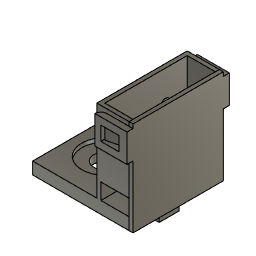
bumper_end (Autodesk Fusion 360 design; units mm, degrees)
Autodesk Fusion 360 part; units mm, degrees
sketch "Sketch1" plane through (0, 0, 0) normal (0, 0, 1) x (1, 0, 0) in component "Halterung"
  line L0 (0, 0) -> (24, 0)
  line L1 (24, 0) -> (24, 20)
  line L2 (24, 20) -> (0, 20)
  line L3 (0, 20) -> (0, 0)
  dimension "d1" = 20
  dimension "d2" = 24
  constraint horizontal L0
  constraint vertical L1
  constraint horizontal L2
  constraint vertical L3
  constraint coincident L0.start L3.end
  measures "d1" distance of L0.start L2.end
  measures "d2" distance of L0.start L0.end
extrude "Extrude1" add sketch "Sketch1" along normal blind 3 makes body 1 in component "Halterung"
sketch "Anbohrung" plane through (0, 0, 3) normal (0, 0, 1) x (-1, 0, 0) in component "Halterung"
  line L0 (0, -20) -> (0, 0)
  line L1 (0, 0) -> (-24, 0)
  line L2 (-24, 0) -> (-24, -20)
  line L3 (-24, -20) -> (0, -20)
  circle A0 centre (-8, -10) radius 5.75
  dimension "d5" = 11.5
  dimension "d6" = 10
  dimension "d21" = 8
  dimension "d22" = 2.25
  measures "d5" diameter of A0
  measures "d6" distance of L3 A0.centre
  measures "d21" distance of L0 A0.centre
  measures "d22" distance of L0 A0
extrude "Extrude2" cut sketch "Anbohrung" against normal blind 1 contours A0 bodies 1 in component "Halterung"
sketch "Bohrloch" plane through (0, 0, 2) normal (0, 0, 1) x (-1, 0, 0) in component "Halterung"
  circle A0 centre (-8, -10) radius 2.75
  circle A1 centre (-8, -10) radius 5.75
  dimension "d10" = 5.5
  constraint concentric A0 A1
  measures "d10" diameter of A0
extrude "Extrude3" cut sketch "Bohrloch" against normal up to surface (2 mm away) contours A0 bodies 1 in component "Halterung"
sketch "Horizontale Halterung" plane through (0, 0, 0) normal (0, 0, -1) x (1, 0, 0) in component "Halterung"
  circle A0 centre (8, -10) radius 2.75
  line L0 (0, 0) -> (0, -20)
  line L1 (0, -20) -> (24, -20)
  line L2 (24, -20) -> (24, 0)
  line L3 (24, 0) -> (0, 0)
  line L4 (24, -7.5) -> (21, -7.5)
  line L5 (24, -12.5) -> (24, -7.5)
  line L6 (21, -12.5) -> (24, -12.5)
  line L7 (21, -7.5) -> (21, -12.5)
  dimension "d44" = 3
  dimension "d45" = 5
  dimension "d46" = 7.5
  constraint collinear L2 L5
  constraint equal L5 L7
  constraint equal L4 L6
  measures "d44" distance of L4.start L4.end
  measures "d45" distance of L4.end L6.start
  measures "d46" distance of L3 L4
extrude "Extrude4" add sketch "Horizontale Halterung" along normal blind 2 contours L2 L4 L5 L6 L7 bodies 1 in component "Halterung"
sketch "Haltearm" plane through (0, 0, 3) normal (0, 0, 1) x (-1, 0, 0) in component "Halterung"
  line L0 (0, -20) -> (0, 0)
  line L1 (0, 0) -> (-24, 0)
  line L2 (-24, 0) -> (-24, -20)
  line L3 (-24, -20) -> (0, -20)
  line L4 (-24, -20) -> (-16, -20)
  line L5 (-16, -20) -> (-16, 0)
  line L6 (-16, 0) -> (-24, 0)
  line L7 (-24, 0) -> (-24, -20)
  circle A0 centre (-8, -10) radius 5.75
  dimension "d18" = 8
  constraint horizontal L4
  constraint vertical L5
  constraint horizontal L6
  constraint vertical L7
  constraint coincident L2.end L3.start
  measures "d18" distance of L2.end L4.end
extrude "Extrude6" add sketch "Haltearm" along normal blind 20.5 contours L1 L2 L3 L4 L5 L6 L7 bodies 1 in component "Halterung"
sketch "Hoehenerweiterung" plane through (0, 20, 0) normal (0, 1, 0) x (-1, 0, 0) in component "Halterung"
  line L0 (-24, 0) -> (0, 0)
  line L1 (0, 0) -> (0, 3)
  line L2 (0, 3) -> (-16, 3)
  line L3 (-16, 3) -> (-16, 23.5)
  line L4 (-16, 23.5) -> (-24, 23.5)
  line L5 (-24, 23.5) -> (-24, 0)
  line L6 (-16, 23.5) -> (-24, 23.5)
  line L7 (-24, 23.5) -> (-24, 0)
  line L8 (-24, 0) -> (-16, 0)
  line L9 (-16, 0) -> (-16, 23.5)
  constraint horizontal L6
  constraint vertical L7
  constraint horizontal L8
  constraint vertical L9
  constraint coincident L0.start L5.end
  constraint coincident L3.end L4.start
extrude "Extrude7" add sketch "Hoehenerweiterung" along normal blind 2.5 contours L0 L3 L4 L5 L6 L7 L8 L9 bodies 1 in component "Halterung"
sketch "Aushoelung" plane through (0, 0, 23.5) normal (0, 0, 1) x (-1, 0, 0) in component "Halterung"
  line L0 (-24, 0) -> (-24, -22.5)
  line L1 (-24, -22.5) -> (-16, -22.5)
  line L2 (-16, -22.5) -> (-16, 0)
  line L3 (-16, 0) -> (-24, 0)
  line L4 (-17, -21.5) -> (-24, -21.5)
  line L5 (-24, -21.5) -> (-24, -1)
  line L6 (-24, -1) -> (-17, -1)
  line L7 (-17, -1) -> (-17, -21.5)
  dimension "d27" = 1
  dimension "d28" = 1
  dimension "d29" = 1
  constraint horizontal L4
  constraint vertical L5
  constraint horizontal L6
  constraint vertical L7
  constraint collinear L0 L5
  measures "d27" distance of L1 L4
  measures "d28" distance of L3 L6
  measures "d29" distance of L2 L7
extrude "Extrude8" cut sketch "Aushoelung" against normal up to surface (20.5 mm away) contours L0 L4 L5 L6 L7 bodies 1 in component "Halterung"
sketch "Servoarme" plane through (17, 0, 0) normal (1, 0, 0) x (0, 1, 0) in component "Halterung"
  line L0 (1, 3) -> (21.5, 3)
  line L1 (21.5, 3) -> (21.5, 23.5)
  line L2 (21.5, 23.5) -> (1, 23.5)
  line L3 (1, 23.5) -> (1, 3)
  circle A0 centre (16.1, 15.9) radius 1.1
  circle A1 centre (6.4, 15.9) radius 1.1
  dimension "d32" = 2.2
  dimension "d34" = 4
  dimension "d35" = 4.3
  dimension "d36" = 6.5
  dimension "d37" = 6.5
  dimension "d40" = 7.5
  constraint equal A0 A1
  measures "d32" diameter of A0
  measures "d35" distance of L3 A1
  measures "d36" distance of L2 A1
  measures "d37" distance of L2 A0
  measures "d40" distance of A0 A1
extrude "Extrude9" add sketch "Servoarme" along normal up to surface (7.5 mm away) contours A0 | A1 bodies 1 in component "Halterung"
sketch "Kabeloeffnung" plane through (0, 1, 0) normal (0, 1, 0) x (-1, 0, 0) in component "Halterung"
  line L0 (-24, 3) -> (-17, 3)
  line L1 (-17, 3) -> (-17, 23.5)
  line L2 (-17, 23.5) -> (-24, 23.5)
  line L3 (-24, 23.5) -> (-24, 3)
  line L4 (-24, 3) -> (-17, 3)
  line L5 (-17, 3) -> (-17, 7)
  line L6 (-17, 7) -> (-24, 7)
  line L7 (-24, 7) -> (-24, 3)
  dimension "d41" = 4
  constraint horizontal L4
  constraint vertical L5
  constraint horizontal L6
  constraint vertical L7
  constraint coincident L1 L5.end
  constraint coincident L0.start L3.end
  measures "d41" distance of L0.start L6.end
extrude "Extrude10" cut sketch "Kabeloeffnung" against normal up to surface (1 mm away) contours L0 L1 L3 L4 L5 L6 L7 bodies 1 in component "Halterung"
sketch "Clip" plane through (0, 0, 0) normal (0, -1, 0) x (1, 0, 0) in component "Halterung"
  line L0 (24, 3) -> (17, 3)
  line L1 (17, 3) -> (17, 7)
  line L2 (17, 7) -> (24, 7)
  line L3 (24, 7) -> (24, 23.5)
  line L4 (24, 23.5) -> (16, 23.5)
  line L5 (16, 23.5) -> (16, 3)
  line L6 (16, 3) -> (0, 3)
  line L7 (0, 3) -> (0, 0)
  line L8 (0, 0) -> (24, 0)
  line L9 (24, 0) -> (24, 3)
  line L10 (19, 20.5) -> (23, 20.5)
  line L11 (23, 20.5) -> (23, 17.5)
  line L12 (23, 17.5) -> (19, 17.5)
  line L13 (19, 17.5) -> (19, 20.5)
  dimension "d48" = 3
  dimension "d49" = 3
  dimension "d50" = 1
  dimension "d52" = 4
  constraint horizontal L10
  constraint vertical L11
  constraint horizontal L12
  constraint vertical L13
  measures "d48" distance of L10.end L11.end
  measures "d49" distance of L4 L10
  measures "d50" distance of L3 L11
  measures "d52" distance of L10.start L10.end
extrude "Extrude11" add sketch "Clip" along normal blind 1 contours L10 L11 L12 L13 bodies 1 in component "Halterung"
chamfer "Chamfer1" distance 4 distance2 1 1 edges at (23, -1, 19) measured on face at (21.6667, -1, 18.5) on bodies 1 in component "Halterung"
sketch "Clip (1)" plane through (0, 22.5, 0) normal (0, 1, 0) x (-1, 0, 0) in component "Halterung"
  line L0 (-16, 0) -> (-16, 23.5)
  line L1 (-16, 23.5) -> (-24, 23.5)
  line L2 (-24, 23.5) -> (-24, 0)
  line L3 (-24, 0) -> (-16, 0)
  line L4 (-23, 20.5) -> (-19, 20.5)
  line L5 (-19, 20.5) -> (-19, 17.5)
  line L6 (-19, 17.5) -> (-23, 17.5)
  line L7 (-23, 17.5) -> (-23, 20.5)
  dimension "d59" = 3
  dimension "d60" = 3
  dimension "d71" = 4
  dimension "d72" = 1
  constraint horizontal L4
  constraint vertical L5
  constraint horizontal L6
  constraint vertical L7
  measures "d59" distance of L4.end L5.end
  measures "d60" distance of L1 L4
  measures "d71" distance of L4.start L4.end
  measures "d72" distance of L2 L7
extrude "Extrude12" add sketch "Clip (1)" along normal blind 1 contours L4 L5 L6 L7 bodies 1 in component "Halterung"
chamfer "Chamfer2" distance 4 distance2 1 1 edges at (23, 23.5, 19) measured on face at (21.6667, 23.5, 19.5) on bodies 1 in component "Halterung"
sketch "Klappe" plane through (24, 0, 0) normal (1, 0, 0) x (0, 1, 0) in component "Klappe"
  line L0 (21.5, 3) -> (0, 3)
  line L1 (0, 3) -> (0, 0)
  line L2 (0, 0) -> (7.5, 0)
  line L3 (7.5, 0) -> (7.5, -2)
  line L4 (7.5, -2) -> (12.5, -2)
  line L5 (12.5, -2) -> (12.5, 0)
  line L6 (12.5, 0) -> (22.5, 0)
  line L7 (22.5, 0) -> (22.5, 23.5)
  line L8 (22.5, 23.5) -> (21.5, 23.5)
  line L9 (21.5, 23.5) -> (21.5, 3)
  line L10 (0, 0) -> (22.5, 0)
  line L11 (22.5, 0) -> (22.5, 23.5)
  line L12 (22.5, 23.5) -> (0, 23.5)
  line L13 (0, 23.5) -> (0, 0)
  constraint horizontal L10
  constraint vertical L11
  constraint horizontal L12
  constraint vertical L13
  constraint coincident L7.end L8.start
  constraint coincident L1.end L2.start
extrude "Extrude1'" add sketch "Klappe" along normal blind 1 separate body contours L0 L1 L2 L6 L7 L8 L9 L10 L11 L12 L13 | L0 L9 L12 L13 makes body 2 in component "Klappe"
extrude "Extrude13" [suppressed] in component "Halterung"
extrude "Extrude2'" cut 2 faces at (24.5, 6.534, 16.3506) (24.5, 16.4463, 15.8466) along direction (-1, 0, 0) blind 0.5 on bodies 1 bodies 2 in component "Klappe"
sketch "Sketch2" plane through (0, 0, 0) normal (0, -1, 0) x (1, 0, 0) in component "Klappe"
  line L0 (24, 23.5) -> (24, 0)
  line L1 (24, 0) -> (25, 0)
  line L2 (25, 0) -> (25, 23.5)
  line L3 (25, 23.5) -> (24, 23.5)
  line L4 (24, 22.5) -> (25, 22.5)
  line L5 (25, 22.5) -> (25, 15.5)
  line L6 (25, 15.5) -> (24, 15.5)
  line L7 (24, 15.5) -> (24, 22.5)
  dimension "d73" = 1
  dimension "d74" = 7
  constraint horizontal L4
  constraint vertical L5
  constraint horizontal L6
  constraint vertical L7
  constraint coincident L2 L5.end
  constraint coincident L0 L4.start
  measures "d73" distance of L3 L4
  measures "d74" distance of L4.end L5.end
extrude "Extrude3'" add sketch "Sketch2" along normal blind 1.5 contours L0 L2 L4 L5 L6 L7 bodies 2 in component "Klappe"
sketch "Sketch3" plane through (0, 22.5, 0) normal (0, 1, 0) x (-1, 0, 0) in component "Klappe"
  line L0 (-24, 0) -> (-24, 23.5)
  line L1 (-24, 23.5) -> (-25, 23.5)
  line L2 (-25, 23.5) -> (-25, 0)
  line L3 (-25, 0) -> (-24, 0)
  line L4 (-25, 22.5) -> (-24, 22.5)
  line L5 (-24, 22.5) -> (-24, 15.5)
  line L6 (-24, 15.5) -> (-25, 15.5)
  line L7 (-25, 15.5) -> (-25, 22.5)
  dimension "d77" = 1
  dimension "d78" = 7
  constraint horizontal L4
  constraint vertical L5
  constraint horizontal L6
  constraint vertical L7
  constraint coincident L0 L5.end
  constraint coincident L2 L4.start
  measures "d77" distance of L1 L4
  measures "d78" distance of L4.start L6.end
extrude "Extrude4'" add sketch "Sketch3" along normal blind 1.5 contours L0 L2 L4 L5 L6 L7 bodies 2 in component "Klappe"
sketch "Sketch4" plane through (24, 0, 0) normal (-1, 0, 0) x (0, -1, 0) in component "Klappe"
  circle A0 centre (-6.4, 15.9) radius 1.1
  circle A1 centre (-16.1, 15.9) radius 1.1
  line L0 (0, 22.5) -> (0, 23.5)
  line L1 (0, 23.5) -> (-22.5, 23.5)
  line L2 (-22.5, 23.5) -> (-22.5, 22.5)
  line L3 (-22.5, 22.5) -> (-24, 22.5)
  line L4 (-24, 22.5) -> (-24, 15.5)
  line L5 (-24, 15.5) -> (-22.5, 15.5)
  line L6 (-22.5, 15.5) -> (-22.5, 0)
  line L7 (-22.5, 0) -> (0, 0)
  line L8 (0, 0) -> (0, 15.5)
  line L9 (0, 15.5) -> (1.5, 15.5)
  line L10 (1.5, 15.5) -> (1.5, 22.5)
  line L11 (1.5, 22.5) -> (0, 22.5)
  line L12 (-24, 22.5) -> (-22.5, 22.5)
  line L13 (-22.5, 22.5) -> (-22.5, 15.5)
  line L14 (-22.5, 15.5) -> (-24, 15.5)
  line L15 (-24, 15.5) -> (-24, 22.5)
  line L16 (0, 22.5) -> (1.5, 22.5)
  line L17 (1.5, 22.5) -> (1.5, 15.5)
  line L18 (1.5, 15.5) -> (0, 15.5)
  line L19 (0, 15.5) -> (0, 22.5)
  constraint horizontal L12
  constraint vertical L13
  constraint horizontal L14
  constraint vertical L15
  constraint coincident L5.end L6.start
  constraint coincident L3.end L4.start
  constraint horizontal L16
  constraint vertical L17
  constraint horizontal L18
  constraint vertical L19
  constraint coincident L9.end L10.start
  constraint coincident L0.start L11.end
extrude "Extrude5" add sketch "Sketch4" along normal blind 7 contours L9 L10 L11 L16 L17 L18 L19 | L3 L4 L5 L12 L13 L14 L15 bodies 2 in component "Klappe"
sketch "Sketch5" plane through (0, 24, 0) normal (0, 1, 0) x (-1, 0, 0) in component "Klappe"
  line L0 (-25, 15.5) -> (-17, 15.5)
  line L1 (-17, 15.5) -> (-17, 22.5)
  line L2 (-17, 22.5) -> (-25, 22.5)
  line L3 (-25, 22.5) -> (-25, 15.5)
  line L4 (-18.5, 20.75) -> (-23, 20.75)
  line L5 (-23, 20.75) -> (-23, 17.25)
  line L6 (-23, 17.25) -> (-18.5, 17.25)
  line L7 (-18.5, 17.25) -> (-18.5, 20.75)
  dimension "d83" = 3.5
  dimension "d84" = 4.5
  dimension "d85" = 1.75
  dimension "d97" = 2
  constraint horizontal L4
  constraint vertical L5
  constraint horizontal L6
  constraint vertical L7
  measures "d83" distance of L4.start L6.end
  measures "d84" distance of L4.start L4.end
  measures "d85" distance of L2 L4
  measures "d97" distance of L3 L5
extrude "Extrude6'" cut sketch "Sketch5" against normal up to surface (1.5 mm away) contours L4 L5 L6 L7 bodies 2 in component "Klappe"
sketch "Sketch6" plane through (0, -1.5, 0) normal (0, -1, 0) x (1, 0, 0) in component "Klappe"
  line L0 (17, 15.5) -> (25, 15.5)
  line L1 (25, 15.5) -> (25, 22.5)
  line L2 (25, 22.5) -> (17, 22.5)
  line L3 (17, 22.5) -> (17, 15.5)
  line L4 (18.5, 20.75) -> (23, 20.75)
  line L5 (23, 20.75) -> (23, 17.25)
  line L6 (23, 17.25) -> (18.5, 17.25)
  line L7 (18.5, 17.25) -> (18.5, 20.75)
  dimension "d89" = 3.5
  dimension "d90" = 4.5
  dimension "d91" = 1.75
  dimension "d98" = 2
  constraint horizontal L4
  constraint vertical L5
  constraint horizontal L6
  constraint vertical L7
  measures "d89" distance of L4.start L6.end
  measures "d90" distance of L4.start L4.end
  measures "d91" distance of L2 L4
  measures "d98" distance of L1 L5
extrude "Extrude7'" cut sketch "Sketch6" against normal up to surface (1.5 mm away) contours L4 L5 L6 L7 bodies 2 in component "Klappe"
fillet "Fillet1" radius 1.5 1 edges at (17, 0, 19) on bodies 2 in component "Klappe"
fillet "Fillet2" radius 1.5 1 edges at (17, 22.5, 19) on bodies 2 in component "Klappe"
component "Halterung" placed x (1, 0, 0) y (0, 1, 0) z (0, 0, 1) at (0, 0, 0)
component "Klappe" placed x (1, 0, 0) y (0, 1, 0) z (0, 0, 1) at (0, 0, 0)
